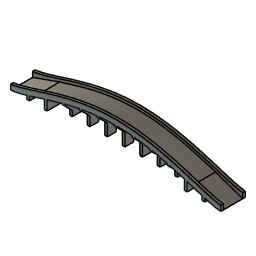
BRIDGE DESIGN v3 (Autodesk Fusion 360 design; units mm, degrees)
Autodesk Fusion 360 part; units mm, degrees
(part 1 of 2)
sketch "Sketch1" plane through (0, 0, 0) normal (0, 1, 0) x (1, 0, 0)
  line L0 (0, 0) -> (73152, 0)
  line L1 (36576, 0) -> (36576, -7620)
  line L2 (7620, 0) -> (7620, -1828.8)
  line L3 (65532, 0) -> (65532, -1828.8)
  spline S0 degree 5 poles (0, 0) (268.5102, -14.4894) (858.3224, -71.4215) (1901.4099, -240.6673) (3610.2762, -634.8152) (6277.6072, -1399.3041) (9467.0595, -2403.3551) (13147.8997, -3572.6656) (17267.153, -4795.7631) (21755.6962, -5944.1158) (26531.6057, -6887.2732) (31503.9734, -7509.9937) (36576, -7728.8755) (41648.0266, -7509.9937) (46620.3943, -6887.2731) (51396.3038, -5944.1157) (55884.8469, -4795.7631) (60004.1003, -3572.6656) (63684.9405, -2403.355) (66874.3928, -1399.304) (69541.7238, -634.8152) (71250.5901, -240.6672) (72293.6776, -71.4215) (72883.4898, -14.4894) (73152, 0) knots 0 0 0 0 0 0 0.05 0.1 0.15 0.2 0.25 0.3 0.35 0.4 0.45 0.5 0.55 0.6 0.65 0.7 0.75 0.8 0.85 0.9 0.95 1 1 1 1 1 1
  line L4 (73152, 0) -> (73152, -915.9212)
  line L5 (0, -915.9214) -> (0, 0)
  spline S1 degree 3 poles (0, -915.9214) (131.7492, -924.0422) (275.4349, -936.8365) (430.3385, -954.5737) (631.9807, -977.6627) (852.6407, -1009.1163) (1091.4063, -1049.1642) (1370.8256, -1096.0308) (1675.0543, -1154.6639) (2003.2902, -1225.1108) (2387.7561, -1307.6259) (2805.1777, -1406.3566) (3254.8084, -1520.9556) (3687.7337, -1631.2968) (4150.5377, -1756.3519) (4642.7059, -1895.3887) (5119.4939, -2030.0806) (5623.8516, -2177.9016) (6155.2434, -2337.6984) (6670.0292, -2492.5015) (7210.1951, -2658.5457) (7775.0361, -2834.2338) (8330.1548, -3006.8978) (8909.1057, -3188.8725) (9510.9669, -3378.1364) (10148.4423, -3578.5998) (10811.6233, -3787.2386) (11499.0935, -4001.1016) (12253.9288, -4235.9209) (13038.0471, -4477.0301) (13849.17, -4719.9647) (14744.4423, -4988.1025) (15672.6153, -5258.4504) (16630.1474, -5524.5468) (17641.5513, -5805.6141) (18685.7116, -6081.9109) (19757.9237, -6345.6598) (20734.1814, -6585.8053) (21733.6852, -6815.5271) (22752.5428, -7029.1759) (23672.3537, -7222.0552) (24607.9329, -7401.8264) (25556.2229, -7564.7052) (26436.32, -7715.8712) (27327.3628, -7852.4824) (28226.783, -7971.936) (29075.6964, -8084.6818) (29932.0709, -8182.1394) (30793.661, -8262.5672) (31616.2068, -8339.3503) (32443.505, -8400.6096) (33273.5419, -8445.2917) (34072.167, -8488.2829) (34873.3265, -8515.9256) (35675.1845, -8527.7544) (36468.6127, -8539.4588) (37262.722, -8535.6774) (38055.7128, -8516.4744) (38875.1791, -8496.6303) (39693.4493, -8460.3198) (40508.5709, -8408.1732) (41358.0326, -8353.8297) (42204.0738, -8282.2904) (43044.5396, -8194.8292) (43964.3855, -8099.1075) (44877.5508, -7984.314) (45781.3042, -7852.765) (46738.8463, -7713.3865) (47685.8202, -7555.205) (48619.1182, -7381.6168) (49636.7495, -7192.3432) (50638.1168, -6984.7611) (51619.4148, -6763.9051) (52702.1287, -6520.2238) (53760.4007, -6260.4022) (54789.5022, -5991.7247) (55810.6284, -5725.1294) (56803.0304, -5449.8451) (57762.5492, -5173.0777) (58630.9789, -4922.5844) (59472.4757, -4670.8911) (60284.3228, -4423.1149) (61014.7425, -4200.1904) (61721.1625, -3980.4442) (62401.8892, -3767.2754) (63034.1316, -3569.2893) (63644.2104, -3376.9821) (64231.0271, -3192.6899) (64804.6881, -3012.5293) (65356.1207, -2840.0297) (65884.5378, -2676.9357) (66421.1466, -2511.3132) (66934.0205, -2355.3936) (67422.5755, -2210.5099) (67944.1719, -2055.8277) (68438.0589, -1913.7221) (68903.7226, -1785.2281) (69393.5534, -1650.0656) (69852.1709, -1529.9574) (70278.9957, -1425.5618) (70668.6983, -1330.2457) (71031.9118, -1248.0201) (71368.0153, -1179.0625) (71662.0677, -1118.7324) (71935.3801, -1068.5561) (72187.2367, -1028.4542) (72391.7191, -995.8954) (72582.0606, -969.9782) (72757.5949, -950.525) (72898.8358, -934.8722) (73030.4952, -923.41) (73152, -915.9212) knots 0.00207705 0.00207705 0.00207705 0.00207705 0.01854804 0.01854804 0.01854804 0.03998876 0.03998876 0.03998876 0.06508013 0.06508013 0.06508013 0.09446988 0.09446988 0.09446988 0.12276769 0.12276769 0.12276769 0.1501812 0.1501812 0.1501812 0.17673804 0.17673804 0.17673804 0.20283777 0.20283777 0.20283777 0.2304819 0.2304819 0.2304819 0.26083488 0.26083488 0.26083488 0.29433681 0.29433681 0.29433681 0.3297236 0.3297236 0.3297236 0.36194355 0.36194355 0.36194355 0.39103129 0.39103129 0.39103129 0.41802728 0.41802728 0.41802728 0.44350732 0.44350732 0.44350732 0.46783269 0.46783269 0.46783269 0.4912375 0.4912375 0.4912375 0.51439626 0.51439626 0.51439626 0.53832821 0.53832821 0.53832821 0.56326839 0.56326839 0.56326839 0.59056412 0.59056412 0.59056412 0.6194844 0.6194844 0.6194844 0.65101794 0.65101794 0.65101794 0.68581042 0.68581042 0.68581042 0.72033328 0.72033328 0.72033328 0.75157881 0.75157881 0.75157881 0.77969045 0.77969045 0.77969045 0.80579986 0.80579986 0.80579986 0.83132392 0.83132392 0.83132392 0.85724366 0.85724366 0.85724366 0.88491638 0.88491638 0.88491638 0.91402526 0.91402526 0.91402526 0.94060246 0.94060246 0.94060246 0.96385449 0.96385449 0.96385449 0.98273282 0.98273282 0.98273282 0.99792296 0.99792296 0.99792296 0.99792296
  line L6 (0, 0) -> (6096, 0)
  line L7 (6096, 0) -> (6096, -1365.5174)
  line L8 (6096, 0) -> (12192, 0)
  line L9 (12192, 0) -> (15239.9998, 0)
  line L10 (12192, 0) -> (14630.3998, 0)
  line L11 (12192, 0) -> (14020.7998, 0)
  line L12 (12192, 0) -> (13411.1999, 0)
  line L13 (12192, 0) -> (18288, 0)
  line L14 (12192, 0) -> (12192, -3258.7165)
  line L15 (18288, 0) -> (18288, -5026.7411)
  line L16 (18288, 0) -> (24384, 0)
  line L17 (24384, 0) -> (24384, -6423.1534)
  line L18 (24384, 0) -> (29260.7996, 0)
  line L19 (24384, 0) -> (26624.6392, 0)
  line L20 (24384, 0) -> (28651.1996, 0)
  line L21 (24384, 0) -> (25918.4173, 0)
  line L22 (24384, 0) -> (30480, 0)
  line L23 (30480, 0) -> (30480, -7313.6498)
  line L24 (30480, 0) -> (36576, 0)
  line L25 (6553.2, -908.3174) -> (5638.8, -908.3174)
  line L26 (5638.8, -908.3174) -> (5638.8, -1822.7174)
  line L27 (5638.8, -1822.7174) -> (6553.2, -1822.7174)
  line L28 (6553.2, -1822.7174) -> (6553.2, -908.3174)
  line L29 (6553.2, -908.3174) -> (5638.8, -1822.7174) construction
  line L30 (5638.8, -908.3174) -> (6553.2, -1822.7174) construction
  line L31 (12649.2, -2801.5165) -> (11734.8, -2801.5165)
  line L32 (11734.8, -2801.5165) -> (11734.8, -3715.9165)
  line L33 (11734.8, -3715.9165) -> (12649.2, -3715.9165)
  line L34 (12649.2, -3715.9165) -> (12649.2, -2801.5165)
  line L35 (12649.2, -2801.5165) -> (11734.8, -3715.9165) construction
  line L36 (11734.8, -2801.5165) -> (12649.2, -3715.9165) construction
  line L37 (18745.2, -4569.5411) -> (17830.8, -4569.5411)
  line L38 (17830.8, -4569.5411) -> (17830.8, -5483.9411)
  line L39 (17830.8, -5483.9411) -> (18745.2, -5483.9411)
  line L40 (18745.2, -5483.9411) -> (18745.2, -4569.5411)
  line L41 (18745.2, -4569.5411) -> (17830.8, -5483.9411) construction
  line L42 (17830.8, -4569.5411) -> (18745.2, -5483.9411) construction
  line L43 (24841.2, -5965.9534) -> (23926.8, -5965.9534)
  line L44 (23926.8, -5965.9534) -> (23926.8, -6880.3534)
  line L45 (23926.8, -6880.3534) -> (24841.2, -6880.3534)
  line L46 (24841.2, -6880.3534) -> (24841.2, -5965.9534)
  line L47 (24841.2, -5965.9534) -> (23926.8, -6880.3534) construction
  line L48 (23926.8, -5965.9534) -> (24841.2, -6880.3534) construction
  line L49 (30937.2, -6856.4498) -> (30022.8, -6856.4498)
  line L50 (30022.8, -6856.4498) -> (30022.8, -7770.8498)
  line L51 (30022.8, -7770.8498) -> (30937.2, -7770.8498)
  line L52 (30937.2, -7770.8498) -> (30937.2, -6856.4498)
  line L53 (30937.2, -6856.4498) -> (30022.8, -7770.8498) construction
  line L54 (30022.8, -6856.4498) -> (30937.2, -7770.8498) construction
  line L55 (37033.2, -7162.8) -> (36118.8, -7162.8)
  line L56 (36118.8, -7162.8) -> (36118.8, -8077.2)
  line L57 (36118.8, -8077.2) -> (37033.2, -8077.2)
  line L58 (37033.2, -8077.2) -> (37033.2, -7162.8)
  line L59 (37033.2, -7162.8) -> (36118.8, -8077.2) construction
  line L60 (36118.8, -7162.8) -> (37033.2, -8077.2) construction
  line L61 (67513.2, -1822.7174) -> (66598.8, -1822.7174)
  line L62 (67513.2, -908.3174) -> (67513.2, -1822.7174)
  line L63 (66598.8, -908.3174) -> (67513.2, -908.3174)
  line L64 (66598.8, -1822.7174) -> (66598.8, -908.3174)
  line L65 (61417.2, -2801.5165) -> (61417.2, -3715.9165)
  line L66 (61417.2, -3715.9165) -> (60502.8, -3715.9165)
  line L67 (60502.8, -3715.9165) -> (60502.8, -2801.5165)
  line L68 (60502.8, -2801.5165) -> (61417.2, -2801.5165)
  line L69 (55321.2, -5483.9411) -> (54406.8, -5483.9411)
  line L70 (54406.8, -5483.9411) -> (54406.8, -4569.5411)
  line L71 (54406.8, -4569.5411) -> (55321.2, -4569.5411)
  line L72 (55321.2, -4569.5411) -> (55321.2, -5483.9411)
  line L73 (49225.2, -6880.3534) -> (48310.8, -6880.3534)
  line L74 (48310.8, -6880.3534) -> (48310.8, -5965.9534)
  line L75 (48310.8, -5965.9534) -> (49225.2, -5965.9534)
  line L76 (49225.2, -5965.9534) -> (49225.2, -6880.3534)
  line L77 (43129.2, -7770.8498) -> (42214.8, -7770.8498)
  line L78 (42214.8, -7770.8498) -> (42214.8, -6856.4498)
  line L79 (42214.8, -6856.4498) -> (43129.2, -6856.4498)
  line L80 (43129.2, -6856.4498) -> (43129.2, -7770.8498)
  point P0 (6096, -1365.5174)
  point P1 (12192, -3258.7165)
  point P2 (18288, -5026.7411)
  point P3 (24384, -6423.1534)
  point P4 (30480, -7313.6498)
  point P5 (36576, -7620)
  dimension "d1" = 73152
  dimension "d2" = 7620
  dimension "d3" = 7620
  dimension "d4" = 1828.8
  dimension "d5" = 7620
  dimension "d7" = 6096
  dimension "d8" = 6096
  dimension "d9" = 6096
  dimension "d10" = 6096
  dimension "d11" = 6096
  dimension "d12" = 914.4
  dimension "d13" = 914.4
  dimension "d14" = 914.4
  dimension "d15" = 914.4
  dimension "d16" = 914.4
  dimension "d17" = 914.4
  dimension "d18" = 914.4
  dimension "d19" = 914.4
  dimension "d20" = 914.4
  dimension "d21" = 914.4
  dimension "d22" = 914.4
  dimension "d23" = 914.4
  constraint coincident L0.start S0.start
  constraint horizontal L0
  constraint midpoint L0 L1.start
  constraint perpendicular L0 L1
  constraint coincident L0 L2.start
  constraint perpendicular L0 L2
  constraint coincident L0 L3.start
  constraint perpendicular L0 L3
  constraint perpendicular L0 L4
  constraint perpendicular L0 L5
  constraint perpendicular L5 L6
  constraint coincident S0 P0
  constraint perpendicular L0 L7
  constraint perpendicular L7 L8
  constraint coincident L0 L9.end
  constraint parallel L0 L9
  constraint coincident L9 L10.end
  constraint coincident L0 L11.end
  constraint midpoint L10 L12.end
  constraint parallel L10 L13
  constraint coincident S0 P1
  constraint perpendicular L9 L14
  constraint coincident S0 P2
  constraint perpendicular L13 L15
  constraint perpendicular L15 L16
  constraint coincident S0 P3
  constraint perpendicular L16 L17
  constraint coincident L0 L18.end
  constraint perpendicular L17 L18
  constraint coincident L0 L19.end
  constraint coincident L0 L20.end
  constraint perpendicular L17 L20
  constraint coincident L19 L21.end
  constraint perpendicular L17 L22
  constraint coincident S0 P4
  constraint perpendicular L0 L23
  constraint horizontal L25
  constraint perpendicular L25 L26
  constraint parallel L25 L27
  constraint parallel L26 L28
  constraint coincident L29 P0
  constraint coincident L30 P0
  constraint coincident P0 L7.end
  constraint horizontal L31
  constraint perpendicular L31 L32
  constraint parallel L31 L33
  constraint parallel L32 L34
  constraint coincident L35 P1
  constraint coincident L36 P1
  constraint coincident P1 L14.end
  constraint horizontal L37
  constraint perpendicular L37 L38
  constraint parallel L37 L39
  constraint parallel L38 L40
  constraint coincident L41 P2
  constraint coincident L42 P2
  constraint coincident P2 L15.end
  constraint horizontal L43
  constraint perpendicular L43 L44
  constraint parallel L43 L45
  constraint parallel L44 L46
  constraint coincident L47 P3
  constraint coincident L48 P3
  constraint coincident P3 L17.end
  constraint horizontal L49
  constraint perpendicular L49 L50
  constraint parallel L49 L51
  constraint parallel L50 L52
  constraint coincident L53 P4
  constraint coincident L54 P4
  constraint coincident P4 L23.end
  constraint horizontal L55
  constraint perpendicular L55 L56
  constraint parallel L55 L57
  constraint parallel L56 L58
  constraint coincident L59 P5
  constraint coincident L60 P5
  constraint coincident P5 L1.end
  constraint symmetric L1 L25.start L63.start
  constraint symmetric L1 L25.end L62.start
  constraint symmetric L1 L26.end L61.start
  constraint symmetric L1 L27.end L61.end
  constraint symmetric L1 L31.start L67.end
  constraint symmetric L1 L31.end L65.start
  constraint symmetric L1 L32.end L65.end
  constraint symmetric L1 L33.end L66.end
  constraint symmetric L1 L37.start L70.end
  constraint symmetric L1 L37.end L71.end
  constraint symmetric L1 L38.end L69.start
  constraint symmetric L1 L39.end L69.end
  constraint symmetric L1 L43.start L74.end
  constraint symmetric L1 L43.end L75.end
  constraint symmetric L1 L44.end L73.start
  constraint symmetric L1 L45.end L73.end
  constraint symmetric L1 L49.start L78.end
  constraint symmetric L1 L49.end L79.end
  constraint symmetric L1 L50.end L77.start
  constraint symmetric L1 L51.end L77.end
  measures "d1" distance of L0.start L0.end
  measures "d2" distance of L1.start P5
  measures "d3" distance of L0.start L2
  measures "d4" distance of L3.start L3.end
  measures "d5" distance of L0.end L3
  measures "d7" distance of L0.start L6.end
  measures "d8" distance of L6.end L8.end
  measures "d9" distance of L8.end L13.end
  measures "d10" distance of L13.end L16.end
  measures "d11" distance of L16.end L22.end
  measures "d12" distance of L26.end L27.end
  measures "d13" distance of L25.end L26.end
  measures "d14" distance of L32.end L33.end
  measures "d15" distance of L31.end L32.end
  measures "d16" distance of L38.end L39.end
  measures "d17" distance of L37.end L38.end
  measures "d18" distance of L44.end L45.end
  measures "d19" distance of L43.end L44.end
  measures "d20" distance of L50.end L51.end
  measures "d21" distance of L49.end L50.end
  measures "d22" distance of L56.end L57.end
  measures "d23" distance of L55.end L56.end
extrude "Extrude1" add sketch "Sketch1" along normal blind 8534.4 contours S0 L4 L5 S1 L26 L27 L28 L32 L33 L34 L38 L39 L40 L44 L45 L46 L50 L51 L52 L56 L57 L58 L61 L62 L64 L65 L66 L67 L69 L70 L72 L73 L74 L76 L77 L78 L80 | S0 L7 L25 L26 | S0 L26 L27 L28 | S0 L7 L25 L28 | S0 L14 L31 L34 | S0 L14 L31 L32 | S0 L32 L33 L34 | S0 L61 L62 L64 | S0 L62 L63 L64 | L1 S0 L55 L58 | L1 S0 L55 L56 | S0 L65 L66 L67 | S0 L65 L67 L68 | S0 L15 L37 L38 | S0 L38 L39 L40 | S0 L23 L49 L52 | S0 L23 L49 L50 | S0 L56 L57 L58 | S0 L15 L37 L40 | S0 L50 L51 L52 | S0 L69 L70 L72 | S0 L70 L71 L72 | S0 L78 L79 L80 | S0 L77 L78 L80 | S0 L17 L43 L46 | S0 L17 L43 L44 | S0 L44 L45 L46 | S0 L73 L74 L76 | S0 L74 L75 L76
sketch "Sketch2" plane through (0, 0, 0) normal (0, 0, 1) x (1, 0, 0)
  line L0 (0, 8534.3999) -> (6096, 8534.3999)
  line L1 (6096, 8534.3999) -> (6096, 4267.1999)
  line L2 (6553.2, 5791.1999) -> (5638.8, 5791.1999)
  line L3 (5638.8, 5791.1999) -> (5638.8, 2743.1999)
  line L4 (5638.8, 2743.1999) -> (6553.2, 2743.1999)
  line L5 (6553.2, 2743.1999) -> (6553.2, 5791.1999)
  line L6 (6553.2, 5791.1999) -> (5638.8, 2743.1999) construction
  line L7 (5638.8, 5791.1999) -> (6553.2, 2743.1999) construction
  line L8 (11734.8, 2743.1999) -> (12649.2, 2743.1999)
  line L9 (12649.2, 2743.1999) -> (12649.2, 5791.1999)
  line L10 (12649.2, 5791.1999) -> (11734.8, 5791.1999)
  line L11 (11734.8, 5791.1999) -> (11734.8, 2743.1999)
  line L12 (17830.8, 2743.1999) -> (18745.2, 2743.1999)
  line L13 (18745.2, 2743.1999) -> (18745.2, 5791.1999)
  line L14 (18745.2, 5791.1999) -> (17830.8, 5791.1999)
  line L15 (17830.8, 5791.1999) -> (17830.8, 2743.1999)
  line L16 (23926.8, 2743.1999) -> (24841.2, 2743.1999)
  line L17 (24841.2, 2743.1999) -> (24841.2, 5791.1999)
  line L18 (24841.2, 5791.1999) -> (23926.8, 5791.1999)
  line L19 (23926.8, 5791.1999) -> (23926.8, 2743.1999)
  line L20 (30022.8, 2743.1999) -> (30937.2, 2743.1999)
  line L21 (30937.2, 2743.1999) -> (30937.2, 5791.1999)
  line L22 (30937.2, 5791.1999) -> (30022.8, 5791.1999)
  line L23 (30022.8, 5791.1999) -> (30022.8, 2743.1999)
  line L24 (36118.8, 2743.1999) -> (37033.2, 2743.1999)
  line L25 (37033.2, 2743.1999) -> (37033.2, 5791.1999)
  line L26 (37033.2, 5791.1999) -> (36118.8, 5791.1999)
  line L27 (36118.8, 5791.1999) -> (36118.8, 2743.1999)
  line L28 (42214.8, 2743.1999) -> (43129.2, 2743.1999)
  line L29 (43129.2, 2743.1999) -> (43129.2, 5791.1999)
  line L30 (43129.2, 5791.1999) -> (42214.8, 5791.1999)
  line L31 (42214.8, 5791.1999) -> (42214.8, 2743.1999)
  line L32 (48310.8, 2743.1999) -> (49225.2, 2743.1999)
  line L33 (49225.2, 2743.1999) -> (49225.2, 5791.1999)
  line L34 (49225.2, 5791.1999) -> (48310.8, 5791.1999)
  line L35 (48310.8, 5791.1999) -> (48310.8, 2743.1999)
  line L36 (54406.8, 2743.1999) -> (55321.2, 2743.1999)
  line L37 (55321.2, 2743.1999) -> (55321.2, 5791.1999)
  line L38 (55321.2, 5791.1999) -> (54406.8, 5791.1999)
  line L39 (54406.8, 5791.1999) -> (54406.8, 2743.1999)
  line L40 (60502.8, 2743.1999) -> (61417.2, 2743.1999)
  line L41 (61417.2, 2743.1999) -> (61417.2, 5791.1999)
  line L42 (61417.2, 5791.1999) -> (60502.8, 5791.1999)
  line L43 (60502.8, 5791.1999) -> (60502.8, 2743.1999)
  line L44 (66598.8, 2743.1999) -> (67513.2, 2743.1999)
  line L45 (67513.2, 2743.1999) -> (67513.2, 5791.1999)
  line L46 (67513.2, 5791.1999) -> (66598.8, 5791.1999)
  line L47 (66598.8, 5791.1999) -> (66598.8, 2743.1999)
  point P0 (6096, 4267.1999)
  dimension "d26" = 6096
  dimension "d27" = 4267.2
  dimension "d28" = 914.4
  dimension "d29" = 3048
  dimension "d32" = 6096
  dimension "d33" = 0
  constraint horizontal L0
  constraint perpendicular L0 L1
  constraint horizontal L2
  constraint perpendicular L2 L3
  constraint parallel L2 L4
  constraint parallel L3 L5
  constraint coincident L6 P0
  constraint coincident L7 P0
  constraint coincident P0 L1.end
  measures "d26" distance of L0.start L0.end
  measures "d27" distance of L0.end P0
  measures "d28" distance of L3.end L4.end
  measures "d29" distance of L2.end L3.end
extrude "Extrude2" add sketch "Sketch2" along normal blind 14630.4
sketch "Sketch3" plane through (0, 0, 0) normal (0, -1, 0) x (1, 0, 0)
  line L0 (37033.2, 7162.8) -> (37033.2, 7618.2618)
  spline S0 degree 5 poles (37033.2, 7618.2618) (37954.428, 7611.2576) (38994.877, 7583.4187) (40033.2545, 7533.1642) (41067.7592, 7461.1483) (42096.6164, 7368.4857) (42214.8, 7357.5637) knots 0.504515 0.504515 0.504515 0.504515 0.504515 0.504515 0.55 0.555907 0.555907 0.555907 0.555907 0.555907 0.555907
  line L1 (42214.8, 7357.5637) -> (42214.8, 6856.4498)
  line L2 (42214.8, 6856.4498) -> (43129.2, 6856.4498)
  line L3 (43129.2, 6856.4498) -> (43129.2, 7266.4285)
  spline S1 degree 5 poles (43129.2, 7266.4285) (43825.0016, 7192.0589) (44874.7874, 7065.4477) (45916.0925, 6918.7228) (46947.0193, 6753.6294) (47965.7319, 6572.2462) (48310.8, 6508.7421) knots 0.565068 0.565068 0.565068 0.565068 0.565068 0.565068 0.6 0.61801 0.61801 0.61801 0.61801 0.61801 0.61801
  line L4 (48310.8, 6508.7421) -> (48310.8, 5965.9534)
  line L5 (48310.8, 5965.9534) -> (49225.2, 5965.9534)
  line L6 (49225.2, 5965.9534) -> (49225.2, 6334.6951)
  spline S2 degree 5 poles (49225.2, 6334.6951) (49650.278, 6251.1311) (50716.0208, 6033.9204) (51765.1865, 5801.4676) (52795.65, 5556.643) (53805.408, 5302.5237) (54406.8, 5146.4697) knots 0.627601 0.627601 0.627601 0.627601 0.627601 0.627601 0.65 0.684088 0.684088 0.684088 0.684088 0.684088 0.684088
  line L7 (54406.8, 5146.4697) -> (54406.8, 4569.5411)
  line L8 (54406.8, 4569.5411) -> (55321.2, 4569.5411)
  line L9 (55321.2, 4569.5411) -> (55321.2, 4904.8773)
  spline S3 degree 5 poles (55321.2, 4904.8773) (55415.9174, 4879.4147) (56375.9101, 4620.2188) (57446.8471, 4318.2729) (58486.5091, 4013.3921) (59492.5544, 3709.9309) (60382.2634, 3436.8803) (60502.8, 3399.8046) knots 0.69454 0.69454 0.69454 0.69454 0.69454 0.69454 0.7 0.75 0.757877 0.757877 0.757877 0.757877 0.757877 0.757877
  line L10 (60502.8, 3399.8046) -> (60502.8, 2801.5165)
  line L11 (60502.8, 2801.5165) -> (61417.2, 2801.5165)
  line L12 (61417.2, 2801.5165) -> (61417.2, 3116.8006)
  spline S4 degree 5 poles (61417.2, 3116.8006) (61863.0996, 2978.034) (62994.1286, 2623.9389) (64068.7047, 2284.2309) (65083.813, 1965.3744) (66037.5097, 1672.043) (66598.8, 1502.5993) knots 0.770001 0.770001 0.770001 0.770001 0.770001 0.770001 0.8 0.847529 0.847529 0.847529 0.847529 0.847529 0.847529
  line L13 (66598.8, 1502.5993) -> (66598.8, 908.3174)
  line L14 (66598.8, 908.3174) -> (67513.2, 908.3174)
  line L15 (67513.2, 908.3174) -> (67513.2, 1230.5462)
  spline S5 degree 5 poles (67513.2, 1230.5462) (67920.4439, 1111.3723) (68851.899, 844.6352) (70197.072, 484.2345) (71344.206, 225.4776) (72293.6776, 71.4215) (72883.4898, 14.4894) (73152, 0) knots 0.863462 0.863462 0.863462 0.863462 0.863462 0.863462 0.9 0.95 1 1 1 1 1 1
  line L16 (73152, 0) -> (73152, 915.9212)
  spline S6 degree 3 poles (0, 915.9214) (131.7492, 924.0422) (275.4349, 936.8365) (430.3385, 954.5737) (631.9807, 977.6627) (852.6407, 1009.1163) (1091.4063, 1049.1642) (1370.8256, 1096.0308) (1675.0543, 1154.6639) (2003.2902, 1225.1108) (2387.7561, 1307.6259) (2805.1777, 1406.3566) (3254.8084, 1520.9556) (3687.7337, 1631.2968) (4150.5377, 1756.3519) (4642.7059, 1895.3887) (5119.4939, 2030.0806) (5623.8516, 2177.9016) (6155.2434, 2337.6984) (6670.0292, 2492.5015) (7210.1951, 2658.5457) (7775.0361, 2834.2338) (8330.1548, 3006.8978) (8909.1057, 3188.8725) (9510.9669, 3378.1364) (10148.4423, 3578.5998) (10811.6233, 3787.2386) (11499.0935, 4001.1016) (12253.9288, 4235.9209) (13038.0471, 4477.0301) (13849.17, 4719.9647) (14744.4423, 4988.1025) (15672.6153, 5258.4504) (16630.1474, 5524.5468) (17641.5513, 5805.6141) (18685.7116, 6081.9109) (19757.9237, 6345.6598) (20734.1814, 6585.8053) (21733.6852, 6815.5271) (22752.5428, 7029.1759) (23672.3537, 7222.0552) (24607.9329, 7401.8264) (25556.2229, 7564.7052) (26436.32, 7715.8712) (27327.3628, 7852.4824) (28226.783, 7971.936) (29075.6964, 8084.6818) (29932.0709, 8182.1394) (30793.661, 8262.5672) (31616.2068, 8339.3503) (32443.505, 8400.6096) (33273.5419, 8445.2917) (34072.167, 8488.2829) (34873.3265, 8515.9256) (35675.1845, 8527.7544) (36468.6127, 8539.4588) (37262.722, 8535.6774) (38055.7128, 8516.4744) (38875.1791, 8496.6303) (39693.4493, 8460.3198) (40508.5709, 8408.1732) (41358.0326, 8353.8297) (42204.0738, 8282.2904) (43044.5396, 8194.8292) (43964.3855, 8099.1075) (44877.5508, 7984.314) (45781.3042, 7852.765) (46738.8463, 7713.3865) (47685.8202, 7555.205) (48619.1182, 7381.6168) (49636.7495, 7192.3432) (50638.1168, 6984.7611) (51619.4148, 6763.9051) (52702.1287, 6520.2238) (53760.4007, 6260.4022) (54789.5022, 5991.7247) (55810.6284, 5725.1294) (56803.0304, 5449.8451) (57762.5492, 5173.0777) (58630.9789, 4922.5844) (59472.4757, 4670.8911) (60284.3228, 4423.1149) (61014.7425, 4200.1904) (61721.1625, 3980.4442) (62401.8892, 3767.2754) (63034.1316, 3569.2893) (63644.2104, 3376.9821) (64231.0271, 3192.6899) (64804.6881, 3012.5293) (65356.1207, 2840.0297) (65884.5378, 2676.9357) (66421.1466, 2511.3132) (66934.0205, 2355.3936) (67422.5755, 2210.5099) (67944.1719, 2055.8277) (68438.0589, 1913.7221) (68903.7226, 1785.2281) (69393.5534, 1650.0656) (69852.1709, 1529.9574) (70278.9957, 1425.5618) (70668.6983, 1330.2457) (71031.9118, 1248.0201) (71368.0153, 1179.0625) (71662.0677, 1118.7324) (71935.3801, 1068.5561) (72187.2367, 1028.4542) (72391.7191, 995.8954) (72582.0606, 969.9782) (72757.5949, 950.525) (72898.8358, 934.8722) (73030.4952, 923.41) (73152, 915.9212) knots 0.00207705 0.00207705 0.00207705 0.00207705 0.01854804 0.01854804 0.01854804 0.03998876 0.03998876 0.03998876 0.06508013 0.06508013 0.06508013 0.09446988 0.09446988 0.09446988 0.12276769 0.12276769 0.12276769 0.1501812 0.1501812 0.1501812 0.17673804 0.17673804 0.17673804 0.20283777 0.20283777 0.20283777 0.2304819 0.2304819 0.2304819 0.26083488 0.26083488 0.26083488 0.29433681 0.29433681 0.29433681 0.3297236 0.3297236 0.3297236 0.36194355 0.36194355 0.36194355 0.39103129 0.39103129 0.39103129 0.41802728 0.41802728 0.41802728 0.44350732 0.44350732 0.44350732 0.46783269 0.46783269 0.46783269 0.4912375 0.4912375 0.4912375 0.51439626 0.51439626 0.51439626 0.53832821 0.53832821 0.53832821 0.56326839 0.56326839 0.56326839 0.59056412 0.59056412 0.59056412 0.6194844 0.6194844 0.6194844 0.65101794 0.65101794 0.65101794 0.68581042 0.68581042 0.68581042 0.72033328 0.72033328 0.72033328 0.75157881 0.75157881 0.75157881 0.77969045 0.77969045 0.77969045 0.80579986 0.80579986 0.80579986 0.83132392 0.83132392 0.83132392 0.85724366 0.85724366 0.85724366 0.88491638 0.88491638 0.88491638 0.91402526 0.91402526 0.91402526 0.94060246 0.94060246 0.94060246 0.96385449 0.96385449 0.96385449 0.98273282 0.98273282 0.98273282 0.99792296 0.99792296 0.99792296 0.99792296
  line L17 (0, 915.9214) -> (0, 0)
  spline S7 degree 5 poles (0, 0) (268.5102, 14.4894) (858.3224, 71.4215) (1807.794, 225.4776) (2954.928, 484.2346) (4300.101, 844.6352) (5231.5561, 1111.3723) (5638.8, 1230.5463) knots 0 0 0 0 0 0 0.05 0.1 0.136538 0.136538 0.136538 0.136538 0.136538 0.136538
  line L18 (5638.8, 1230.5463) -> (5638.8, 908.3174)
  line L19 (5638.8, 908.3174) -> (6553.2, 908.3174)
  line L20 (6553.2, 908.3174) -> (6553.2, 1502.5994)
  spline S8 degree 5 poles (6553.2, 1502.5994) (7114.4903, 1672.043) (8068.187, 1965.3744) (9083.2952, 2284.231) (10157.8714, 2623.9389) (11288.9004, 2978.0341) (11734.8, 3116.8007) knots 0.152471 0.152471 0.152471 0.152471 0.152471 0.152471 0.2 0.229999 0.229999 0.229999 0.229999 0.229999 0.229999
  line L21 (11734.8, 3116.8007) -> (11734.8, 2801.5165)
  line L22 (11734.8, 2801.5165) -> (12649.2, 2801.5165)
  line L23 (12649.2, 2801.5165) -> (12649.2, 3399.8047)
  spline S9 degree 5 poles (12649.2, 3399.8047) (12769.7366, 3436.8803) (13659.4456, 3709.931) (14665.4909, 4013.3922) (15705.1529, 4318.2729) (16776.0899, 4620.2189) (17736.0826, 4879.4148) (17830.8, 4904.8773) knots 0.242123 0.242123 0.242123 0.242123 0.242123 0.242123 0.25 0.3 0.30546 0.30546 0.30546 0.30546 0.30546 0.30546
  line L24 (17830.8, 4904.8773) -> (17830.8, 4569.5411)
  line L25 (17830.8, 4569.5411) -> (18745.2, 4569.5411)
  line L26 (18745.2, 4569.5411) -> (18745.2, 5146.4697)
  spline S10 degree 5 poles (18745.2, 5146.4697) (19346.592, 5302.5237) (20356.35, 5556.6431) (21386.8135, 5801.4676) (22435.9792, 6033.9205) (23501.722, 6251.1311) (23926.8, 6334.6951) knots 0.315912 0.315912 0.315912 0.315912 0.315912 0.315912 0.35 0.372399 0.372399 0.372399 0.372399 0.372399 0.372399
  line L27 (23926.8, 6334.6951) -> (23926.8, 5965.9534)
  line L28 (23926.8, 5965.9534) -> (24841.2, 5965.9534)
  line L29 (24841.2, 5965.9534) -> (24841.2, 6508.7422)
  spline S11 degree 5 poles (24841.2, 6508.7422) (25186.2681, 6572.2462) (26204.9807, 6753.6295) (27235.9075, 6918.7228) (28277.2126, 7065.4477) (29326.9984, 7192.0589) (30022.8, 7266.4285) knots 0.38199 0.38199 0.38199 0.38199 0.38199 0.38199 0.4 0.434932 0.434932 0.434932 0.434932 0.434932 0.434932
  line L30 (30022.8, 7266.4285) -> (30022.8, 6856.4498)
  line L31 (30022.8, 6856.4498) -> (30937.2, 6856.4498)
  line L32 (30937.2, 6856.4498) -> (30937.2, 7357.5637)
  spline S12 degree 5 poles (30937.2, 7357.5637) (31055.3836, 7368.4857) (32084.2408, 7461.1483) (33118.7455, 7533.1642) (34157.123, 7583.4188) (35197.572, 7611.2576) (36118.8, 7618.2618) knots 0.444093 0.444093 0.444093 0.444093 0.444093 0.444093 0.45 0.495485 0.495485 0.495485 0.495485 0.495485 0.495485
  line L33 (36118.8, 7618.2618) -> (36118.8, 7162.8)
  line L34 (36118.8, 7162.8) -> (37033.2, 7162.8)
  line L35 (0, 915.9214) -> (914.4, 17373.6005)
  line L36 (914.4, 17373.6005) -> (70898.5123, 18667.449)
  line L37 (70898.5123, 18667.449) -> (73152, 915.9212)
  constraint coincident S6.start L17.start
  constraint coincident L16.end S6.end
extrude "Extrude3" cut sketch "Sketch3" against normal blind 21945.6 contours S6 L35 L36 L37
extrude "Extrude4" add 4 faces at (67208.4, 2743.1999, 605.5449) (60807.6, 2743.1999, 933.8388) (12192, 2743.1999, 933.8388) (6096, 2743.1999, 302.7725) along direction (0, -1, 0) up to surface end surface through (0, 0, 0) normal (0, -1, 0) offset 0
extrude "Extrude5" add 4 faces at (66903.6, 5791.1999, 605.5449) (60807.6, 5791.1999, 1867.6777) (6248.4, 5791.1999, 302.7725) (12344.4, 5791.1999, 1867.6777) along direction (0, 1, 0) up to surface end surface through (0, 8534.4, 0) normal (0, 1, 0) offset 0
chamfer "Chamfer1" distance 2712.72 angle 45 14 edges at (54864, 5791.1999, 4569.5411) (48768, 5791.1999, 5965.9534) (42672, 5791.1999, 6856.4498) (36576, 5791.1999, 7162.8) (30480, 5791.1999, 6856.4498) (24384, 5791.1999, 5965.9534) (18288, 5791.1999, 4569.5411) (18288, 2743.1999, 4569.5411) (24384, 2743.1999, 5965.9534) (30480, 2743.1999, 6856.4498) (36576, 2743.1999, 7162.8) (42672, 2743.1999, 6856.4498) (48768, 2743.1999, 5965.9534) (54864, 2743.1999, 4569.5411)
sketch "Sketch4" plane through (0, 8534.4, 0) normal (0, 1, 0) x (-1, 0, 0)
  line L0 (-37033.2, 7618.2618) -> (-37033.2, 7162.8)
  line L1 (-37033.2, 7162.8) -> (-36118.8, 7162.8)
  line L2 (-36118.8, 7162.8) -> (-36118.8, 7618.2618)
  spline S0 degree 5 poles (-36118.8, 7618.2618) (-35197.572, 7611.2576) (-34157.123, 7583.4188) (-33118.7455, 7533.1642) (-32084.2408, 7461.1483) (-31055.3836, 7368.4857) (-30937.2, 7357.5637) knots -0.495485 -0.495485 -0.495485 -0.495485 -0.495485 -0.495485 -0.45 -0.444093 -0.444093 -0.444093 -0.444093 -0.444093 -0.444093
  line L3 (-30937.2, 7357.5637) -> (-30937.2, 6856.4498)
  line L4 (-30937.2, 6856.4498) -> (-30022.8, 6856.4498)
  line L5 (-30022.8, 6856.4498) -> (-30022.8, 7266.4285)
  spline S1 degree 5 poles (-30022.8, 7266.4285) (-29326.9984, 7192.0589) (-28277.2126, 7065.4477) (-27235.9075, 6918.7228) (-26204.9807, 6753.6295) (-25186.2681, 6572.2462) (-24841.2, 6508.7422) knots -0.434932 -0.434932 -0.434932 -0.434932 -0.434932 -0.434932 -0.4 -0.38199 -0.38199 -0.38199 -0.38199 -0.38199 -0.38199
  line L6 (-24841.2, 6508.7422) -> (-24841.2, 5965.9534)
  line L7 (-24841.2, 5965.9534) -> (-23926.8, 5965.9534)
  line L8 (-23926.8, 5965.9534) -> (-23926.8, 6334.6951)
  spline S2 degree 5 poles (-23926.8, 6334.6951) (-23501.722, 6251.1311) (-22435.9792, 6033.9205) (-21386.8135, 5801.4676) (-20356.35, 5556.6431) (-19346.592, 5302.5237) (-18745.2, 5146.4697) knots -0.372399 -0.372399 -0.372399 -0.372399 -0.372399 -0.372399 -0.35 -0.315912 -0.315912 -0.315912 -0.315912 -0.315912 -0.315912
  line L9 (-18745.2, 5146.4697) -> (-18745.2, 4569.5411)
  line L10 (-18745.2, 4569.5411) -> (-17830.8, 4569.5411)
  line L11 (-17830.8, 4569.5411) -> (-17830.8, 4904.8773)
  spline S3 degree 5 poles (-17830.8, 4904.8773) (-17736.0826, 4879.4148) (-16776.0899, 4620.2189) (-15705.1529, 4318.2729) (-14665.4909, 4013.3922) (-13659.4456, 3709.931) (-12769.7366, 3436.8803) (-12649.2, 3399.8047) knots -0.30546 -0.30546 -0.30546 -0.30546 -0.30546 -0.30546 -0.3 -0.25 -0.242123 -0.242123 -0.242123 -0.242123 -0.242123 -0.242123
  line L12 (-12649.2, 3399.8047) -> (-12649.2, 0)
  line L13 (-12649.2, 0) -> (-11734.8, 0)
  line L14 (-11734.8, 0) -> (-11734.8, 3116.8007)
  spline S4 degree 5 poles (-11734.8, 3116.8007) (-11288.9004, 2978.0341) (-10157.8714, 2623.9389) (-9083.2952, 2284.231) (-8068.187, 1965.3744) (-7114.4903, 1672.043) (-6553.2, 1502.5994) knots -0.229999 -0.229999 -0.229999 -0.229999 -0.229999 -0.229999 -0.2 -0.152471 -0.152471 -0.152471 -0.152471 -0.152471 -0.152471
  line L15 (-6553.2, 1502.5994) -> (-6553.2, 0)
  line L16 (-6553.2, 0) -> (-5638.8, 0)
  line L17 (-5638.8, 0) -> (-5638.8, 1230.5463)
  spline S5 degree 5 poles (-5638.8, 1230.5463) (-5231.5561, 1111.3723) (-4300.101, 844.6352) (-2954.928, 484.2346) (-1807.794, 225.4776) (-858.3224, 71.4215) (-268.5102, 14.4894) (0, 0) knots -0.136538 -0.136538 -0.136538 -0.136538 -0.136538 -0.136538 -0.1 -0.05 0 0 0 0 0 0
  line L18 (0, 0) -> (0, 915.9214)
  spline S6 degree 3 poles (0, 915.9214) (-131.7492, 924.0422) (-275.4349, 936.8365) (-430.3385, 954.5737) (-631.9807, 977.6627) (-852.6407, 1009.1163) (-1091.4063, 1049.1642) (-1370.8256, 1096.0308) (-1675.0543, 1154.6639) (-2003.2902, 1225.1108) (-2387.7561, 1307.6259) (-2805.1777, 1406.3566) (-3254.8084, 1520.9556) (-3687.7337, 1631.2968) (-4150.5377, 1756.3519) (-4642.7059, 1895.3887) (-5119.4939, 2030.0806) (-5623.8516, 2177.9016) (-6155.2434, 2337.6984) (-6670.0292, 2492.5015) (-7210.1951, 2658.5457) (-7775.0361, 2834.2338) (-8330.1548, 3006.8978) (-8909.1057, 3188.8725) (-9510.9669, 3378.1364) (-10148.4423, 3578.5998) (-10811.6233, 3787.2386) (-11499.0935, 4001.1016) (-12253.9288, 4235.9209) (-13038.0471, 4477.0301) (-13849.17, 4719.9647) (-14744.4423, 4988.1025) (-15672.6153, 5258.4504) (-16630.1474, 5524.5468) (-17641.5513, 5805.6141) (-18685.7116, 6081.9109) (-19757.9237, 6345.6598) (-20734.1814, 6585.8053) (-21733.6852, 6815.5271) (-22752.5428, 7029.1759) (-23672.3537, 7222.0552) (-24607.9329, 7401.8264) (-25556.2229, 7564.7052) (-26436.32, 7715.8712) (-27327.3628, 7852.4824) (-28226.783, 7971.936) (-29075.6964, 8084.6818) (-29932.0709, 8182.1394) (-30793.661, 8262.5672) (-31616.2068, 8339.3503) (-32443.505, 8400.6096) (-33273.5419, 8445.2917) (-34072.167, 8488.2829) (-34873.3265, 8515.9256) (-35675.1845, 8527.7544) (-36468.6127, 8539.4588) (-37262.722, 8535.6774) (-38055.7128, 8516.4744) (-38875.1791, 8496.6303) (-39693.4493, 8460.3198) (-40508.5709, 8408.1732) (-41358.0326, 8353.8297) (-42204.0738, 8282.2904) (-43044.5396, 8194.8292) (-43964.3855, 8099.1075) (-44877.5508, 7984.314) (-45781.3042, 7852.765) (-46738.8463, 7713.3865) (-47685.8202, 7555.205) (-48619.1182, 7381.6168) (-49636.7495, 7192.3432) (-50638.1168, 6984.7611) (-51619.4148, 6763.9051) (-52702.1287, 6520.2238) (-53760.4007, 6260.4022) (-54789.5022, 5991.7247) (-55810.6284, 5725.1294) (-56803.0304, 5449.8451) (-57762.5492, 5173.0777) (-58630.9789, 4922.5844) (-59472.4757, 4670.8911) (-60284.3228, 4423.1149) (-61014.7425, 4200.1904) (-61721.1625, 3980.4442) (-62401.8892, 3767.2754) (-63034.1316, 3569.2893) (-63644.2104, 3376.9821) (-64231.0271, 3192.6899) (-64804.6881, 3012.5293) (-65356.1207, 2840.0297) (-65884.5378, 2676.9357) (-66421.1466, 2511.3132) (-66934.0205, 2355.3936) (-67422.5755, 2210.5099) (-67944.1719, 2055.8277) (-68438.0589, 1913.7221) (-68903.7226, 1785.2281) (-69393.5534, 1650.0656) (-69852.1709, 1529.9574) (-70278.9957, 1425.5618) (-70668.6983, 1330.2457) (-71031.9118, 1248.0201) (-71368.0153, 1179.0625) (-71662.0677, 1118.7324) (-71935.3801, 1068.5561) (-72187.2367, 1028.4542) (-72391.7191, 995.8954) (-72582.0606, 969.9782) (-72757.5949, 950.525) (-72898.8358, 934.8722) (-73030.4952, 923.41) (-73152, 915.9212) knots 0.00207705 0.00207705 0.00207705 0.00207705 0.01854804 0.01854804 0.01854804 0.03998876 0.03998876 0.03998876 0.06508013 0.06508013 0.06508013 0.09446988 0.09446988 0.09446988 0.12276769 0.12276769 0.12276769 0.1501812 0.1501812 0.1501812 0.17673804 0.17673804 0.17673804 0.20283777 0.20283777 0.20283777 0.2304819 0.2304819 0.2304819 0.26083488 0.26083488 0.26083488 0.29433681 0.29433681 0.29433681 0.3297236 0.3297236 0.3297236 0.36194355 0.36194355 0.36194355 0.39103129 0.39103129 0.39103129 0.41802728 0.41802728 0.41802728 0.44350732 0.44350732 0.44350732 0.46783269 0.46783269 0.46783269 0.4912375 0.4912375 0.4912375 0.51439626 0.51439626 0.51439626 0.53832821 0.53832821 0.53832821 0.56326839 0.56326839 0.56326839 0.59056412 0.59056412 0.59056412 0.6194844 0.6194844 0.6194844 0.65101794 0.65101794 0.65101794 0.68581042 0.68581042 0.68581042 0.72033328 0.72033328 0.72033328 0.75157881 0.75157881 0.75157881 0.77969045 0.77969045 0.77969045 0.80579986 0.80579986 0.80579986 0.83132392 0.83132392 0.83132392 0.85724366 0.85724366 0.85724366 0.88491638 0.88491638 0.88491638 0.91402526 0.91402526 0.91402526 0.94060246 0.94060246 0.94060246 0.96385449 0.96385449 0.96385449 0.98273282 0.98273282 0.98273282 0.99792296 0.99792296 0.99792296 0.99792296
  line L19 (-73152, 915.9212) -> (-73152, 0)
  spline S7 degree 5 poles (-73152, 0) (-72883.4898, 14.4894) (-72293.6776, 71.4215) (-71344.206, 225.4776) (-70197.072, 484.2345) (-68851.899, 844.6352) (-67920.4439, 1111.3723) (-67513.2, 1230.5462) knots -1 -1 -1 -1 -1 -1 -0.95 -0.9 -0.863462 -0.863462 -0.863462 -0.863462 -0.863462 -0.863462
  line L20 (-67513.2, 1230.5462) -> (-67513.2, 0)
  line L21 (-67513.2, 0) -> (-66598.8, 0)
  line L22 (-66598.8, 0) -> (-66598.8, 1502.5993)
  spline S8 degree 5 poles (-66598.8, 1502.5993) (-66037.5097, 1672.043) (-65083.813, 1965.3744) (-64068.7047, 2284.2309) (-62994.1286, 2623.9389) (-61863.0996, 2978.034) (-61417.2, 3116.8006) knots -0.847529 -0.847529 -0.847529 -0.847529 -0.847529 -0.847529 -0.8 -0.770001 -0.770001 -0.770001 -0.770001 -0.770001 -0.770001
  line L23 (-61417.2, 3116.8006) -> (-61417.2, 0)
  line L24 (-61417.2, 0) -> (-60502.8, 0)
  line L25 (-60502.8, 0) -> (-60502.8, 3399.8046)
  spline S9 degree 5 poles (-60502.8, 3399.8046) (-60382.2634, 3436.8803) (-59492.5544, 3709.9309) (-58486.5091, 4013.3921) (-57446.8471, 4318.2729) (-56375.9101, 4620.2188) (-55415.9174, 4879.4147) (-55321.2, 4904.8773) knots -0.757877 -0.757877 -0.757877 -0.757877 -0.757877 -0.757877 -0.75 -0.7 -0.69454 -0.69454 -0.69454 -0.69454 -0.69454 -0.69454
  line L26 (-55321.2, 4904.8773) -> (-55321.2, 4569.5411)
  line L27 (-55321.2, 4569.5411) -> (-54406.8, 4569.5411)
  line L28 (-54406.8, 4569.5411) -> (-54406.8, 5146.4697)
  spline S10 degree 5 poles (-54406.8, 5146.4697) (-53805.408, 5302.5237) (-52795.65, 5556.643) (-51765.1865, 5801.4676) (-50716.0208, 6033.9204) (-49650.278, 6251.1311) (-49225.2, 6334.6951) knots -0.684088 -0.684088 -0.684088 -0.684088 -0.684088 -0.684088 -0.65 -0.627601 -0.627601 -0.627601 -0.627601 -0.627601 -0.627601
  line L29 (-49225.2, 6334.6951) -> (-49225.2, 5965.9534)
  line L30 (-49225.2, 5965.9534) -> (-48310.8, 5965.9534)
  line L31 (-48310.8, 5965.9534) -> (-48310.8, 6508.7421)
  spline S11 degree 5 poles (-48310.8, 6508.7421) (-47965.7319, 6572.2462) (-46947.0193, 6753.6294) (-45916.0925, 6918.7228) (-44874.7874, 7065.4477) (-43825.0016, 7192.0589) (-43129.2, 7266.4285) knots -0.61801 -0.61801 -0.61801 -0.61801 -0.61801 -0.61801 -0.6 -0.565068 -0.565068 -0.565068 -0.565068 -0.565068 -0.565068
  line L32 (-43129.2, 7266.4285) -> (-43129.2, 6856.4498)
  line L33 (-43129.2, 6856.4498) -> (-42214.8, 6856.4498)
  line L34 (-42214.8, 6856.4498) -> (-42214.8, 7357.5637)
  spline S12 degree 5 poles (-42214.8, 7357.5637) (-42096.6164, 7368.4857) (-41067.7592, 7461.1483) (-40033.2545, 7533.1642) (-38994.877, 7583.4187) (-37954.428, 7611.2576) (-37033.2, 7618.2618) knots -0.555907 -0.555907 -0.555907 -0.555907 -0.555907 -0.555907 -0.55 -0.504515 -0.504515 -0.504515 -0.504515 -0.504515 -0.504515
  line L35 (-68427.6, 19.4625) -> (-68427.6, -914.4)
  line L36 (-68427.6, -914.4) -> (-65684.4, -914.4)
  line L37 (-65684.4, -914.4) -> (-65684.4, 825.1081)
  spline S13 degree 3 poles (-65684.4, 825.1081) (-65379.862, 918.4978) (-65068.0983, 1014.9898) (-64749.2208, 1114.2786) (-64181.0014, 1291.2048) (-63590.1803, 1477.0374) (-62977.6561, 1669.6532) (-62764.9043, 1736.5556) (-62549.5381, 1804.2718) (-62331.6, 1872.7007) knots -0.836785 -0.836785 -0.836785 -0.836785 -0.821947 -0.821947 -0.821947 -0.795507 -0.795507 -0.795507 -0.786323 -0.786323 -0.786323 -0.786323
  line L38 (-62331.6, 1872.7007) -> (-62331.6, -914.4)
  line L39 (-62331.6, -914.4) -> (-59588.4, -914.4)
  line L40 (-59588.4, -914.4) -> (-59588.4, 2723.3632)
  spline S14 degree 3 poles (-59588.4, 2723.3632) (-58966.2425, 2912.7055) (-58327.9952, 3103.779) (-57674.8164, 3294.3308) (-57202.7088, 3432.0587) (-56722.8061, 3569.5102) (-56235.6, 3705.8038) knots -0.749487 -0.749487 -0.749487 -0.749487 -0.72545 -0.72545 -0.72545 -0.708076 -0.708076 -0.708076 -0.708076
  line L41 (-56235.6, 3705.8038) -> (-56235.6, 3655.1411)
  line L42 (-56235.6, 3655.1411) -> (-53492.4, 3655.1411)
  line L43 (-53492.4, 3655.1411) -> (-53492.4, 4436.5293)
  spline S15 degree 3 poles (-53492.4, 4436.5293) (-52744.3829, 4625.0562) (-51982.8657, 4807.6381) (-51209.6335, 4981.586) (-50855.3534, 5061.2855) (-50498.6158, 5139.174) (-50139.6, 5215.0034) knots -0.676302 -0.676302 -0.676302 -0.676302 -0.650928 -0.650928 -0.650928 -0.639302 -0.639302 -0.639302 -0.639302
  line L44 (-50139.6, 5215.0034) -> (-50139.6, 5051.5534)
  line L45 (-50139.6, 5051.5534) -> (-47396.4, 5051.5534)
  line L46 (-47396.4, 5051.5534) -> (-47396.4, 5743.2822)
  spline S16 degree 3 poles (-47396.4, 5743.2822) (-46777.1894, 5850.624) (-46152.8748, 5950.5457) (-45524.3503, 6042.0944) (-45033.1936, 6113.6345) (-44539.4666, 6180.0636) (-44043.6, 6240.983) knots -0.610125 -0.610125 -0.610125 -0.610125 -0.590631 -0.590631 -0.590631 -0.575398 -0.575398 -0.575398 -0.575398
  line L47 (-44043.6, 6240.983) -> (-44043.6, 5942.0498)
  line L48 (-44043.6, 5942.0498) -> (-41300.4, 5942.0498)
  line L49 (-41300.4, 5942.0498) -> (-41300.4, 6518.1784)
  spline S17 degree 3 poles (-41300.4, 6518.1784) (-40730.3632, 6563.1629) (-40158.5941, 6600.3032) (-39585.7282, 6629.2874) (-39040.4981, 6656.8734) (-38494.2745, 6677.0713) (-37947.6, 6689.722) knots -0.5475 -0.5475 -0.5475 -0.5475 -0.530211 -0.530211 -0.530211 -0.513756 -0.513756 -0.513756 -0.513756
  line L50 (-37947.6, 6689.722) -> (-37947.6, 6248.4)
  line L51 (-37947.6, 6248.4) -> (-35204.4, 6248.4)
  line L52 (-35204.4, 6248.4) -> (-35204.4, 6689.722)
  spline S18 degree 3 poles (-35204.4, 6689.722) (-34715.4419, 6678.407) (-34226.8445, 6661.0556) (-33738.9959, 6637.7778) (-33108.3305, 6607.6853) (-32478.9163, 6567.6831) (-31851.6, 6518.1784) knots -0.486244 -0.486244 -0.486244 -0.486244 -0.471526 -0.471526 -0.471526 -0.4525 -0.4525 -0.4525 -0.4525
  line L53 (-31851.6, 6518.1784) -> (-31851.6, 5942.0498)
  line L54 (-31851.6, 5942.0498) -> (-29108.4, 5942.0498)
  line L55 (-29108.4, 5942.0498) -> (-29108.4, 6240.983)
  spline S19 degree 3 poles (-29108.4, 6240.983) (-28553.4099, 6172.8) (-28001.1002, 6097.7139) (-27452.0745, 6016.2876) (-26882.8302, 5931.8627) (-26317.1166, 5840.6226) (-25755.6, 5743.2823) knots -0.424602 -0.424602 -0.424602 -0.424602 -0.407553 -0.407553 -0.407553 -0.389875 -0.389875 -0.389875 -0.389875
  line L56 (-25755.6, 5743.2823) -> (-25755.6, 5051.5534)
  line L57 (-25755.6, 5051.5534) -> (-23012.4, 5051.5534)
  line L58 (-23012.4, 5051.5534) -> (-23012.4, 5215.0035)
  spline S20 degree 3 poles (-23012.4, 5215.0035) (-22349.74, 5075.04) (-21694.8428, 4928.0558) (-21048.8265, 4775.6317) (-20580.9582, 4665.2407) (-20117.7474, 4551.9988) (-19659.6, 4436.5294) knots -0.360698 -0.360698 -0.360698 -0.360698 -0.339239 -0.339239 -0.339239 -0.323698 -0.323698 -0.323698 -0.323698
  line L59 (-19659.6, 4436.5294) -> (-19659.6, 3655.1411)
  line L60 (-19659.6, 3655.1411) -> (-16916.4, 3655.1411)
  line L61 (-16916.4, 3655.1411) -> (-16916.4, 3705.8038)
  spline S21 degree 3 poles (-16916.4, 3705.8038) (-16386.6206, 3557.6006) (-15865.4766, 3408.0283) (-15353.5989, 3258.2196) (-14743.4442, 3079.6486) (-14146.4614, 2900.7465) (-13563.6, 2723.3632) knots -0.291924 -0.291924 -0.291924 -0.291924 -0.273032 -0.273032 -0.273032 -0.250513 -0.250513 -0.250513 -0.250513
  line L62 (-13563.6, 2723.3632) -> (-13563.6, -914.4)
  line L63 (-13563.6, -914.4) -> (-10820.4, -914.4)
  line L64 (-10820.4, -914.4) -> (-10820.4, 1872.7007)
  spline S22 degree 3 poles (-10820.4, 1872.7007) (-10571.1849, 1794.4514) (-10325.3325, 1717.1341) (-10082.9073, 1640.8996) (-9491.1149, 1454.8009) (-8919.7726, 1275.1869) (-8369.69, 1103.9777) (-8062.326, 1008.3129) (-7761.5959, 915.265) (-7467.6, 825.1081) knots -0.213677 -0.213677 -0.213677 -0.213677 -0.203175 -0.203175 -0.203175 -0.177539 -0.177539 -0.177539 -0.163215 -0.163215 -0.163215 -0.163215
  line L65 (-7467.6, 825.1081) -> (-7467.6, -914.4)
  line L66 (-7467.6, -914.4) -> (-4724.4, -914.4)
  line L67 (-4724.4, -914.4) -> (-4724.4, 19.4625)
  spline S23 degree 3 poles (-4724.4, 19.4625) (-4642.2534, -3.1901) (-4560.8649, -25.4582) (-4480.2303, -47.3389) (-4012.5303, -174.252) (-3570.2705, -288.0915) (-3153.1329, -388.2956) (-2759.4567, -482.8639) (-2388.1607, -565.2989) (-2038.5983, -635.3207) (-1726.0742, -697.9234) (-1430.9287, -750.615) (-1152.3168, -793.2043) (-925.4451, -827.8845) (-709.5371, -855.8731) (-503.8303, -876.9668) (-346.5214, -893.0977) (-195.1753, -905.1983) (-49.2713, -913.0716) (271.9525, -930.4055) (593.1762, -947.7394) (914.4, -965.0733) knots -0.114885 -0.114885 -0.114885 -0.114885 -0.110138 -0.110138 -0.110138 -0.082603 -0.082603 -0.082603 -0.056617 -0.056617 -0.056617 -0.033385 -0.033385 -0.033385 -0.014467 -0.014467 -0.014467 0 0 0 0.03589 0.03589 0.03589 0.03589
  line L68 (914.4, -965.0733) -> (914.4, 1775.6946)
  line L69 (0, 915.9214) -> (0, 1832.3275)
  line L70 (-73152, 915.9212) -> (-73152, 1832.3263)
  spline S24 degree 3 poles (914.4, 1775.6946) (628.3518, 1793.3261) (342.3036, 1810.9577) (56.2554, 1828.5892) (-43.0676, 1834.7114) (-153.4958, 1844.1301) (-273.7353, 1857.1739) (-291.0585, 1859.0532) (-308.5861, 1861.0074) (-326.3151, 1863.0375) (-479.0764, 1880.5294) (-647.1897, 1903.7035) (-829.2752, 1932.8039) (-865.6757, 1938.6213) (-902.6363, 1944.6752) (-940.148, 1950.967) (-1172.4521, 1989.9311) (-1426.2036, 2038.0838) (-1700.0051, 2095.5113) (-1736.7781, 2103.2242) (-1773.9136, 2111.1042) (-1811.4087, 2119.1515) (-2149.1783, 2191.6446) (-2516.4342, 2277.7962) (-2911.7712, 2377.3368) (-2950.5676, 2387.1052) (-2989.6348, 2397.0026) (-3028.9718, 2407.0285) (-3452.8022, 2515.0517) (-3908.227, 2638.0862) (-4394.1182, 2775.3498) (-4864.8206, 2908.3225) (-5364.4024, 3054.731) (-5891.9192, 3213.3625) (-6402.9517, 3367.037) (-6940.4642, 3532.2599) (-7503.4553, 3707.3725) (-8056.7593, 3879.472) (-8634.8769, 4061.1831) (-9236.6636, 4250.4237) (-9874.0626, 4450.863) (-10538.2048, 4659.8056) (-11227.4751, 4874.2286) (-11984.293, 5109.6647) (-12771.5571, 5351.7467) (-13586.8176, 5595.9206) (-14486.6654, 5865.4287) (-15420.7167, 6137.5) (-16385.3154, 6405.5602) (-17404.1983, 6688.7059) (-18457.1688, 6967.3511) (-19539.5054, 7233.5905) (-20524.9923, 7476.0062) (-21534.7301, 7708.095) (-22564.8798, 7924.1116) (-23494.8893, 8119.1295) (-24441.4025, 8301.0131) (-25401.4318, 8465.9083) (-26292.4266, 8618.9461) (-27194.9144, 8757.321) (-28106.3969, 8878.3766) (-28966.6976, 8992.6347) (-29834.8495, 9091.4393) (-30708.673, 9173.0091) (-31542.8995, 9250.8826) (-32382.1229, 9313.0292) (-33224.3895, 9358.3697) (-34034.7833, 9401.9944) (-34847.8127, 9430.0487) (-35661.6969, 9442.0549) (-36467.0271, 9453.9349) (-37272.9931, 9450.0967) (-38077.8493, 9430.6064) (-38909.5757, 9410.4654) (-39739.9071, 9373.617) (-40566.9494, 9320.7078) (-41428.8321, 9265.5697) (-42286.9404, 9193.0048) (-43139.1835, 9104.318) (-44071.9194, 9007.2549) (-44997.414, 8890.9029) (-45913.015, 8757.6294) (-46883.1061, 8616.4244) (-47841.8844, 8456.2597) (-48786.3238, 8280.5994) (-49816.0992, 8089.067) (-50828.6317, 7879.1559) (-51820.1921, 7655.9902) (-52914.2203, 7409.7625) (-53982.551, 7147.4536) (-55020.4908, 6876.4685) (-56050.3711, 6607.5877) (-57050.2709, 6330.2091) (-58015.9706, 6051.6589) (-58889.9847, 5799.5548) (-59736.0247, 5546.4948) (-60551.2435, 5297.6895) (-61284.691, 5073.8409) (-61993.2781, 4853.4172) (-62675.1477, 4639.8905) (-63308.4474, 4441.5734) (-63918.828, 4249.1707) (-64505.0047, 4065.0795) (-65078.038, 3885.1161) (-65628.111, 3713.0444) (-66154.2114, 3550.6653) (-66688.4643, 3385.77) (-67198.2045, 3230.8097) (-67682.5547, 3087.173) (-68199.6614, 2933.8222) (-68688.1152, 2793.2955) (-69146.9497, 2666.686) (-69629.5995, 2533.5049) (-70079.8061, 2415.6345) (-70496.2419, 2313.7799) (-70876.4656, 2220.7823) (-71228.8274, 2141.0663) (-71551.7927, 2074.8042) (-71810.3415, 2021.7583) (-72050.2759, 1977.2916) (-72270.2581, 1941.2895) (-72290.6853, 1937.9464) (-72310.94, 1934.6762) (-72331.0211, 1931.4788) (-72508.0211, 1903.2959) (-72671.7814, 1880.7412) (-72820.9986, 1863.5756) (-72833.5407, 1862.1328) (-72845.9799, 1860.7279) (-72858.315, 1859.3609) (-72963.861, 1847.664) (-73062.0347, 1838.7234) (-73152, 1832.3263) knots -0.03368403 -0.03368403 -0.03368403 -0.03368403 0.00207705 0.00207705 0.00207705 0.01647386 0.01647386 0.01647386 0.01854804 0.01854804 0.01854804 0.03641666 0.03641666 0.03641666 0.03998876 0.03998876 0.03998876 0.06210922 0.06210922 0.06210922 0.06508013 0.06508013 0.06508013 0.09184346 0.09184346 0.09184346 0.09446988 0.09446988 0.09446988 0.12276769 0.12276769 0.12276769 0.1501812 0.1501812 0.1501812 0.17673804 0.17673804 0.17673804 0.20283777 0.20283777 0.20283777 0.2304819 0.2304819 0.2304819 0.26083488 0.26083488 0.26083488 0.29433681 0.29433681 0.29433681 0.3297236 0.3297236 0.3297236 0.36194355 0.36194355 0.36194355 0.39103129 0.39103129 0.39103129 0.41802728 0.41802728 0.41802728 0.44350732 0.44350732 0.44350732 0.46783269 0.46783269 0.46783269 0.4912375 0.4912375 0.4912375 0.51439626 0.51439626 0.51439626 0.53832821 0.53832821 0.53832821 0.56326839 0.56326839 0.56326839 0.59056412 0.59056412 0.59056412 0.6194844 0.6194844 0.6194844 0.65101794 0.65101794 0.65101794 0.68581042 0.68581042 0.68581042 0.72033328 0.72033328 0.72033328 0.75157881 0.75157881 0.75157881 0.77969045 0.77969045 0.77969045 0.80579986 0.80579986 0.80579986 0.83132392 0.83132392 0.83132392 0.85724366 0.85724366 0.85724366 0.88491638 0.88491638 0.88491638 0.91402526 0.91402526 0.91402526 0.94060246 0.94060246 0.94060246 0.9618788 0.9618788 0.9618788 0.96385449 0.96385449 0.96385449 0.98126907 0.98126907 0.98126907 0.98273282 0.98273282 0.98273282 0.99526002 0.99526002 0.99526002 0.99526002
  constraint coincident L18.end S6.start